Autodesk Fusion 360 part; units mm, degrees
note: some values were not read from the file. Chosen so that the rebuilt part matches the saved one: which bodies a step acts on. Set by a fixed rule: which sketch regions a step uses.
(part 3 of 3)
sketch "Sketch8" plane through (0, 0, -71) normal (0, 0, 1) x (-1, 0, 0) in component "DipCase"
  line L0 (23.45, 45.575) -> (23.45, 72.575)
  arc A0 (18.95, 77.075) -> (23.45, 72.575) centre (23.45, 77.075) ccw
  line L1 (18.95, 77.075) -> (-57.05, 77.075)
  arc A1 (-61.55, 72.575) -> (-57.05, 77.075) centre (-61.55, 77.075) ccw
  line L2 (-61.55, 72.575) -> (-61.55, 66.575)
  line L3 (-61.55, 66.575) -> (-62.84, 66.575)
  line L4 (-62.84, 66.575) -> (-62.84, 51.575)
  line L5 (-62.84, 51.575) -> (-61.55, 51.575)
  line L6 (-61.55, 51.575) -> (-61.55, 45.575)
  arc A2 (-57.05, 41.075) -> (-61.55, 45.575) centre (-61.55, 41.075) ccw
  line L7 (-57.05, 41.075) -> (18.95, 41.075)
  arc A3 (23.45, 45.575) -> (18.95, 41.075) centre (23.45, 41.075) ccw
  line L8 (-61.55, 66.575) -> (-61.55, 51.575)
  constraint coincident L2.end L3.start
  constraint coincident L5.end L6.start
extrude "Extrude7''" add sketch "Sketch8" along normal blind 30 contours L3 L4 L5 L8 bodies 5 in component "DipCase"
sketch "Sketch9" plane through (61.55, 0, 0) normal (-1, 0, 0) x (0, -1, 0) in component "DipCase"
  line L0 (45.575, -71) -> (72.575, -71)
  line L1 (72.575, -71) -> (72.575, -5.6)
  line L2 (72.575, -5.6) -> (66.575, -5.6)
  line L3 (66.575, -5.6) -> (66.575, -41)
  line L4 (66.575, -41) -> (51.575, -41)
  line L5 (51.575, -41) -> (51.575, -5.6)
  line L6 (51.575, -5.6) -> (45.575, -5.6)
  line L7 (45.575, -5.6) -> (45.575, -71)
  line L8 (51.575, -41) -> (45.575, -41)
  line L9 (45.575, -41) -> (66.575, -41)
  line L10 (66.575, -41) -> (72.575, -41)
  line L11 (59.075, -41) -> (59.075, -71) construction
  line L12 (48.075, -51) -> (70.075, -51)
  line L13 (70.075, -51) -> (70.075, -61)
  line L14 (70.075, -61) -> (48.075, -61)
  line L15 (48.075, -61) -> (48.075, -51)
  line L16 (48.075, -51) -> (70.075, -61) construction
  line L17 (70.075, -51) -> (48.075, -61) construction
  line L18 (54.075, -54) -> (64.075, -54)
  line L19 (64.075, -54) -> (64.075, -58)
  line L20 (64.075, -58) -> (54.075, -58)
  line L21 (54.075, -58) -> (54.075, -54)
  line L22 (54.075, -54) -> (64.075, -58) construction
  line L23 (64.075, -54) -> (54.075, -58) construction
  point P0 (59.075, -56)
  point P1 (59.075, -56)
  point P2 (59.075, -56)
  dimension "d257" = 22
  dimension "d258" = 10
  dimension "d259" = 10
  dimension "d260" = 4
  constraint coincident L4.end L5.start
  constraint coincident L7 L8.end
  constraint perpendicular L7 L8
  constraint coincident L3.end L4.start
  constraint coincident L1 L10.end
  constraint perpendicular L1 L10
  constraint midpoint L4 L11.start
  constraint midpoint L0 L11.end
  constraint midpoint L11 P2
  constraint horizontal L12
  constraint perpendicular L12 L13
  constraint parallel L12 L14
  constraint parallel L13 L15
  constraint coincident L16 P2
  constraint coincident L17 P2
  constraint coincident P2 P1
  constraint horizontal L18
  constraint perpendicular L18 L19
  constraint parallel L18 L20
  constraint parallel L19 L21
  constraint coincident L22 P2
  constraint coincident L23 P2
  measures "d257" distance of L13.end L14.end
  measures "d258" distance of L12.end L13.end
  measures "d259" distance of L19.end L20.end
  measures "d260" distance of L18.end L19.end
extrude "Extrude8''" cut sketch "Sketch9" against normal up to surface (5 mm away) contours L18 L19 L20 L21 bodies 5 in component "DipCase"
extrude "Extrude9'" cut sketch "Sketch9" against normal blind 3 contours L12 L13 L14 L15 bodies 5 in component "DipCase"
sketch "Sketch10" plane through (0, -82.075, 0) normal (0, -1, 0) x (1, 0, 0) in component "DipCase"
  line L0 (45.85, -44.8) -> (-7.75, -44.8)
  line L1 (-7.75, -44.8) -> (-7.75, -36.2)
  line L2 (-7.75, -36.2) -> (45.85, -36.2)
  line L3 (45.85, -36.2) -> (45.85, -44.8)
  line L4 (-25.45, -76) -> (63.55, -76)
  line L5 (63.55, -76) -> (63.55, -5.6)
  line L6 (63.55, -5.6) -> (-25.45, -5.6)
  line L7 (-25.45, -5.6) -> (-25.45, -76)
  line L8 (42.85, -41.8) -> (-4.75, -41.8)
  line L9 (-4.75, -41.8) -> (-4.75, -39.2)
  line L10 (-4.75, -39.2) -> (42.85, -39.2)
  line L11 (42.85, -39.2) -> (42.85, -41.8)
  dimension "d268" = 3
extrude "Extrude11" add sketch "Sketch10" against normal up to surface (5 mm away) contours L0 L1 L2 L3 bodies 5 in component "DipCase"
sketch "Sketch1 (5)" plane through (0, -82.075, 0) normal (0, -1, 0) x (1, 0, 0) in component "BusLegend"
  line L0 (-4.75, -39.2) -> (42.85, -39.2)
  line L1 (42.85, -39.2) -> (42.85, -41.8)
  line L2 (42.85, -41.8) -> (-4.75, -41.8)
  line L3 (-4.75, -41.8) -> (-4.75, -39.2)
  line L4 (-25.45, -76) -> (63.55, -76)
  line L5 (63.55, -76) -> (63.55, -5.6)
  line L6 (63.55, -5.6) -> (-25.45, -5.6)
  line L7 (-25.45, -5.6) -> (-25.45, -76)
  line L8 (-4.75, -39.2) -> (42.85, -39.2)
  line L9 (19.05, -39.2) -> (19.05, -41.8) construction
  line L10 (17.78, -40.5) -> (20.32, -40.5) construction
  line L11 (-9.75, -31.2) -> (47.85, -31.2)
  line L12 (47.85, -31.2) -> (47.85, -38.2)
  line L13 (47.85, -38.2) -> (-9.75, -38.2)
  line L14 (-9.75, -38.2) -> (-9.75, -31.2)
  line L15 (-9.75, -31.2) -> (47.85, -38.2) construction
  line L16 (47.85, -31.2) -> (-9.75, -38.2) construction
  line L17 (19.05, -39.2) -> (19.05, -38.2) construction
  line L18 (-4.75, -39.2) -> (-9.75, -39.2) construction
  line L19 (-9.75, -39.2) -> (-9.75, -38.2) construction
  line L20 (-8.75, -37.7) -> (46.85, -37.7) construction
  line L21 (46.85, -37.7) -> (46.85, -31.7) construction
  line L22 (46.85, -31.7) -> (-8.75, -31.7) construction
  line L23 (-8.75, -31.7) -> (-8.75, -37.7) construction
  line L24 (46.85, -37.7) -> (46.85, -37.7001) construction
  line L25 (-8.75, -31.7) -> (46.85, -37.7) construction
  line L26 (-8.75, -37.7) -> (46.85, -31.7) construction
  line L27 (46.85, -31.7) -> (47.85, -31.7) construction
  point P0 (22.86, -40.5)
  point P1 (25.4, -40.5)
  point P2 (27.94, -40.5)
  point P3 (30.48, -40.5)
  point P4 (33.02, -40.5)
  point P5 (35.56, -40.5)
  point P6 (38.1, -40.5)
  point P7 (40.64, -40.5)
  point P8 (15.24, -40.5)
  point P9 (12.7, -40.5)
  point P10 (10.16, -40.5)
  point P11 (7.62, -40.5)
  point P12 (5.08, -40.5)
  point P13 (2.54, -40.5)
  point P14 (0, -40.5)
  point P15 (-2.54, -40.5)
  point P16 (19.05, -34.7)
  point P17 (19.05, -34.7)
  dimension "d272" = 2.54
  dimension "d275" = 2.54
  dimension "d276" = 0
  dimension "d279" = -2.54
  dimension "d280" = 0
  dimension "d281" = 1
  dimension "d282" = 5
  dimension "d283" = 7
  dimension "d284" = 3
  dimension "d285" = 1
  dimension "d286" = 6
  text T0 "GND | MS----------------LS | 5V" font "Arial" height 3 align centre middle in box 55.6 x 6 at (-8.75, -37.7) x (1, 0) y (0, 1) spacing 1
  constraint midpoint L0 L9.start
  constraint midpoint L2 L9.end
  constraint perpendicular L9 L10
  constraint midpoint L9 L10
  constraint horizontal L11
  constraint perpendicular L11 L12
  constraint parallel L11 L13
  constraint parallel L12 L14
  constraint coincident L15 P17
  constraint coincident L16 P17
  constraint midpoint L13 L17.end
  constraint midpoint L15 P17
  constraint perpendicular L13 L17
  constraint coincident L0.start L3.end
  constraint perpendicular L3 L18
  constraint perpendicular L18 L19
  constraint coincident L20.end
  constraint coincident L21 L24.end
  constraint coincident L22.end
  constraint coincident L20.start
  constraint coincident L21.end
  constraint midpoint L26 P17
  constraint horizontal L22
  constraint coincident P17 P16
  constraint coincident L12 L27.end
  constraint perpendicular L12 L27
  measures "d272" distance of L10.start L10.end
  measures "d281" distance of L9.start L17.end
  measures "d282" distance of L0.start L18.end
  measures "d283" distance of L11.end L12.end
  measures "d285" distance of L21.end L27.end
extrude "Extrude1''''" add sketch "Sketch1 (5)" along normal blind 4 separate body text T0 makes body 6 at (-4.9746, -83.4083, -35.2) makes body 7 at (2.3085, -83.4083, -35.7709) makes body 8 at (9.2968, -82.075, -34.7626) makes body 9 at (12.3692, -84.7417, -34.9292) makes body 10 at (15.5377, -83.4083, -35.2996) makes body 11 at (18.329, -83.4083, -35.2996) makes body 12 at (21.1203, -83.4083, -35.2996) makes body 13 at (23.5343, -84.7417, -34.9292) makes body 14 at (26.7028, -84.7417, -35.2996) makes body 15 at (29.1168, -84.7417, -34.9292) makes body 16 at (33.1005, -83.4083, -35.2) makes body 17 at (36.7532, -82.075, -34.7626) makes body 18 at (46.0391, -83.4083, -34.2) makes body 19 at (39.4688, -83.4083, -35.7709) makes body 20 at (41.6735, -83.4083, -34.2682) makes body 21 at (31.9081, -84.7417, -35.2996) makes body 22 at (30.8897, -83.4083, -35.2996) makes body 23 at (28.0984, -83.4083, -35.2996) makes body 24 at (25.3072, -83.4083, -35.2996) makes body 25 at (22.5159, -83.4083, -35.2996) makes body 26 at (19.7246, -83.4083, -35.2996) makes body 27 at (16.5561, -84.7417, -34.9292) makes body 28 at (13.7649, -84.7417, -34.9292) makes body 29 at (11.3508, -83.4083, -35.2996) makes body 30 at (4.4879, -83.4083, -35.2) makes body 31 at (-1.9439, -83.4083, -35.2) makes body 32 at (-6.4029, -84.7417, -34.6707) in component "BusLegend"
extrude "Extrude2''''" add sketch "Sketch1 (5)" along normal blind 3 contours L11 L12 L13 L14 bodies 6 7 8 9 10 11 12 13 14 15 16 17 18 19 20 21 22 23 24 25 26 27 28 29 30 31 32 in component "BusLegend"
sketch "Sketch2 (5)" plane through (0, -85.075, 0) normal (0, -1, 0) x (1, 0, 0) in component "BusLegend"
  line L0 (-9.75, -38.2) -> (47.85, -38.2)
  line L1 (47.85, -38.2) -> (47.85, -31.2)
  line L2 (47.85, -31.2) -> (-9.75, -31.2)
  line L3 (-9.75, -31.2) -> (-9.75, -38.2)
  line L4 (-6.8265, -35.0233) -> (-6.8265, -34.6714)
  line L5 (-6.8265, -34.6714) -> (-5.5557, -34.6693)
  line L6 (-5.5557, -34.6693) -> (-5.5557, -35.7825)
  spline S0 degree 3 poles (-6.1594, -36.1335) (-6.0463, -36.0845) (-5.9446, -36.0405) (-5.7434, -35.9229) (-5.6496, -35.8527) (-5.5557, -35.7825) knots -0.070377 -0.070377 -0.070377 -0.070377 -0.035159 -0.035159 0 0 0 0
  spline S1 degree 3 poles (-6.7979, -36.2512) (-6.6879, -36.2461) (-6.5797, -36.2412) (-6.3669, -36.2019) (-6.2631, -36.1677) (-6.1594, -36.1335) knots -0.065532 -0.065532 -0.065532 -0.065532 -0.032766 -0.032766 0 0 0 0
  spline S2 degree 3 poles (-7.6011, -36.0619) (-7.4683, -36.1204) (-7.3453, -36.1746) (-7.0773, -36.2371) (-6.9376, -36.2441) (-6.7979, -36.2512) knots -0.083967 -0.083967 -0.083967 -0.083967 -0.041966 -0.041966 0 0 0 0
  spline S3 degree 3 poles (-8.1465, -35.5145) (-8.0768, -35.628) (-8.0081, -35.7401) (-7.8262, -35.9225) (-7.7136, -35.9922) (-7.6011, -36.0619) knots -0.079423 -0.079423 -0.079423 -0.079423 -0.039711 -0.039711 0 0 0 0
  spline S4 degree 3 poles (-8.3306, -34.7143) (-8.3239, -34.8533) (-8.3172, -34.9922) (-8.2565, -35.2593) (-8.2039, -35.3813) (-8.1465, -35.5145) knots -0.086964 -0.086964 -0.086964 -0.086964 -0.043506 -0.043506 0 0 0 0
  spline S5 degree 3 poles (-8.1475, -33.8968) (-8.2025, -34.0303) (-8.2554, -34.1587) (-8.3161, -34.4313) (-8.3234, -34.5728) (-8.3306, -34.7143) knots -0.085018 -0.085018 -0.085018 -0.085018 -0.042505 -0.042505 0 0 0 0
  spline S6 degree 3 poles (-7.6205, -33.333) (-7.7355, -33.4081) (-7.8421, -33.4776) (-8.0172, -33.6662) (-8.0823, -33.7815) (-8.1475, -33.8968) knots -0.079495 -0.079495 -0.079495 -0.079495 -0.039731 -0.039731 0 0 0 0
  spline S7 degree 3 poles (-6.8286, -33.1488) (-6.9664, -33.1551) (-7.1042, -33.1614) (-7.3687, -33.2217) (-7.4868, -33.2739) (-7.6205, -33.333) knots -0.087597 -0.087597 -0.087597 -0.087597 -0.043852 -0.043852 0 0 0 0
  spline S8 degree 3 poles (-6.2402, -33.2542) (-6.3414, -33.2205) (-6.4309, -33.1906) (-6.6274, -33.156) (-6.728, -33.1524) (-6.8286, -33.1488) knots -0.060473 -0.060473 -0.060473 -0.060473 -0.030201 -0.030201 0 0 0 0
  spline S9 degree 3 poles (-5.8279, -33.5479) (-5.8908, -33.4808) (-5.9453, -33.4227) (-6.0835, -33.3254) (-6.1619, -33.2898) (-6.2402, -33.2542) knots -0.051721 -0.051721 -0.051721 -0.051721 -0.025816 -0.025816 0 0 0 0
  spline S10 degree 3 poles (-5.6008, -34.039) (-5.626, -33.9512) (-5.6513, -33.8635) (-5.7263, -33.6986) (-5.772, -33.6309) (-5.8279, -33.5479) knots -0.059807 -0.059807 -0.059807 -0.059807 -0.030023 -0.030023 0 0 0 0
  line L7 (-5.6008, -34.039) -> (-5.9589, -34.1372)
  spline S11 degree 3 poles (-6.1267, -33.7771) (-6.0861, -33.8397) (-6.0546, -33.8883) (-5.9991, -34.0097) (-5.979, -34.0735) (-5.9589, -34.1372) knots -0.040416 -0.040416 -0.040416 -0.040416 -0.020059 -0.020059 0 0 0 0
  spline S12 degree 3 poles (-6.4132, -33.5673) (-6.3586, -33.5931) (-6.304, -33.6189) (-6.2078, -33.6884) (-6.1707, -33.729) (-6.1267, -33.7771) knots -0.039026 -0.039026 -0.039026 -0.039026 -0.019563 -0.019563 0 0 0 0
  spline S13 degree 3 poles (-6.8265, -33.4885) (-6.7556, -33.4913) (-6.6847, -33.4941) (-6.5468, -33.52) (-6.4835, -33.5424) (-6.4132, -33.5673) knots -0.044711 -0.044711 -0.044711 -0.044711 -0.022375 -0.022375 0 0 0 0
  spline S14 degree 3 poles (-7.2972, -33.5714) (-7.2141, -33.5434) (-7.1451, -33.5202) (-6.9876, -33.4933) (-6.9071, -33.4909) (-6.8265, -33.4885) knots -0.048493 -0.048493 -0.048493 -0.048493 -0.024168 -0.024168 0 0 0 0
  spline S15 degree 3 poles (-7.6175, -33.7894) (-7.567, -33.7408) (-7.5233, -33.6988) (-7.416, -33.6265) (-7.3566, -33.599) (-7.2972, -33.5714) knots -0.039361 -0.039361 -0.039361 -0.039361 -0.019646 -0.019646 0 0 0 0
  spline S16 degree 3 poles (-7.8068, -34.0861) (-7.7811, -34.0316) (-7.7564, -33.9791) (-7.6932, -33.8802) (-7.6553, -33.8348) (-7.6175, -33.7894) knots -0.035488 -0.035488 -0.035488 -0.035488 -0.017742 -0.017742 0 0 0 0
  spline S17 degree 3 poles (-7.9214, -34.6898) (-7.9171, -34.5863) (-7.9128, -34.4829) (-7.8749, -34.2815) (-7.8421, -34.1874) (-7.8068, -34.0861) knots -0.064337 -0.064337 -0.064337 -0.064337 -0.032181 -0.032181 0 0 0 0
  spline S18 degree 3 poles (-7.7832, -35.361) (-7.831, -35.2426) (-7.8696, -35.147) (-7.9141, -34.9218) (-7.9177, -34.8058) (-7.9214, -34.6898) knots -0.069971 -0.069971 -0.069971 -0.069971 -0.034827 -0.034827 0 0 0 0
  spline S19 degree 3 poles (-7.3811, -35.7621) (-7.466, -35.7111) (-7.5483, -35.6617) (-7.6821, -35.5278) (-7.7327, -35.4444) (-7.7832, -35.361) knots -0.058521 -0.058521 -0.058521 -0.058521 -0.029259 -0.029259 0 0 0 0
  spline S20 degree 3 poles (-6.8204, -35.893) (-6.9177, -35.8876) (-7.015, -35.8822) (-7.2019, -35.8386) (-7.2912, -35.8005) (-7.3811, -35.7621) knots -0.05867 -0.05867 -0.05867 -0.05867 -0.029335 -0.029335 0 0 0 0
  spline S21 degree 3 poles (-6.317, -35.7938) (-6.3985, -35.8225) (-6.48, -35.8513) (-6.6478, -35.8845) (-6.7329, -35.8887) (-6.8204, -35.893) knots -0.052539 -0.052539 -0.052539 -0.052539 -0.026271 -0.026271 0 0 0 0
  spline S22 degree 3 poles (-5.9445, -35.582) (-6.0094, -35.6308) (-6.0582, -35.6677) (-6.1842, -35.738) (-6.2506, -35.7659) (-6.317, -35.7938) knots -0.043642 -0.043642 -0.043642 -0.043642 -0.0216 -0.0216 0 0 0 0
  line L8 (-5.9445, -35.582) -> (-5.9445, -35.0233)
  line L9 (-5.9445, -35.0233) -> (-6.8265, -35.0233)
  line L10 (4.4879, -36.2) -> (4.4879, -33.2)
  line L11 (4.4879, -33.2) -> (5.0855, -33.2)
  line L12 (5.0855, -33.2) -> (5.7956, -35.3241)
  spline S23 degree 3 poles (5.9388, -35.7682) (5.9122, -35.6833) (5.8933, -35.623) (5.8444, -35.4718) (5.82, -35.398) (5.7956, -35.3241) knots -0.047666 -0.047666 -0.047666 -0.047666 -0.023331 -0.023331 0 0 0 0
  spline S24 degree 3 poles (6.0984, -35.2873) (6.0711, -35.3672) (6.0438, -35.4472) (5.9894, -35.6106) (5.9684, -35.6762) (5.9388, -35.7682) knots -0.056865 -0.056865 -0.056865 -0.056865 -0.028983 -0.028983 0 0 0 0
  line L13 (6.0984, -35.2873) -> (6.8167, -33.2)
  line L14 (6.8167, -33.2) -> (7.3508, -33.2)
  line L15 (7.3508, -33.2) -> (7.3508, -36.2)
  line L16 (7.3508, -36.2) -> (6.9681, -36.2)
  line L17 (6.9681, -36.2) -> (6.9681, -33.6891)
  line L18 (6.9681, -33.6891) -> (6.0964, -36.2)
  line L19 (6.0964, -36.2) -> (5.7383, -36.2)
  line L20 (5.7383, -36.2) -> (4.8706, -33.6461)
  line L21 (4.8706, -33.6461) -> (4.8706, -36.2)
  line L22 (4.8706, -36.2) -> (4.4879, -36.2)
  line L23 (13.3877, -35.2996) -> (13.3877, -34.9292)
  line L24 (13.3877, -34.9292) -> (14.5193, -34.9292)
  line L25 (14.5193, -34.9292) -> (14.5193, -35.2996)
  line L26 (14.5193, -35.2996) -> (13.3877, -35.2996)
  line L27 (18.9702, -35.2996) -> (18.9702, -34.9292)
  line L28 (18.9702, -34.9292) -> (20.1018, -34.9292)
  line L29 (20.1018, -34.9292) -> (20.1018, -35.2996)
  line L30 (20.1018, -35.2996) -> (18.9702, -35.2996)
  line L31 (24.5527, -35.2996) -> (24.5527, -34.9292)
  line L32 (24.5527, -34.9292) -> (25.6844, -34.9292)
  line L33 (25.6844, -34.9292) -> (25.6844, -35.2996)
  line L34 (25.6844, -35.2996) -> (24.5527, -35.2996)
  line L35 (30.1353, -35.2996) -> (30.1353, -34.9292)
  line L36 (30.1353, -34.9292) -> (31.2669, -34.9292)
  line L37 (31.2669, -34.9292) -> (31.2669, -35.2996)
  line L38 (31.2669, -35.2996) -> (30.1353, -35.2996)
  line L39 (34.975, -35.846) -> (34.975, -36.2)
  line L40 (34.975, -36.2) -> (33.1005, -36.2)
  line L41 (35.3126, -35.2362) -> (35.6871, -35.2034)
  line L42 (41.9224, -34.8269) -> (41.5766, -34.7819)
  line L43 (41.5766, -34.7819) -> (41.8672, -33.2409)
  spline S25 degree 3 poles (45.2151, -35.3794) (45.1856, -35.4604) (45.1561, -35.5414) (45.1022, -35.7052) (45.0781, -35.7868) (45.0534, -35.8705) knots -0.052408 -0.052408 -0.052408 -0.052408 -0.026205 -0.026205 0 0 0 0
  line L44 (41.8672, -33.2409) -> (43.359, -33.2409)
  line L45 (43.359, -33.2409) -> (43.359, -33.5929)
  line L46 (43.359, -33.5929) -> (42.1619, -33.5929)
  line L47 (42.1619, -33.5929) -> (42.0002, -34.3992)
  line L48 (39.4688, -37.082) -> (39.4688, -33.1488)
  line L49 (39.4688, -33.1488) -> (39.7901, -33.1488)
  line L50 (39.7901, -33.1488) -> (39.7901, -37.082)
  line L51 (37.6107, -34.0452) -> (37.2301, -34.0738)
  line L52 (25.9484, -35.2996) -> (25.9484, -34.9292)
  line L53 (25.9484, -34.9292) -> (27.08, -34.9292)
  line L54 (27.08, -34.9292) -> (27.08, -35.2996)
  line L55 (27.08, -35.2996) -> (25.9484, -35.2996)
  line L56 (20.3658, -35.2996) -> (20.3658, -34.9292)
  line L57 (20.3658, -34.9292) -> (21.4975, -34.9292)
  line L58 (21.4975, -34.9292) -> (21.4975, -35.2996)
  line L59 (21.4975, -35.2996) -> (20.3658, -35.2996)
  line L60 (14.7833, -35.2996) -> (14.7833, -34.9292)
  line L61 (14.7833, -34.9292) -> (15.9149, -34.9292)
  line L62 (15.9149, -34.9292) -> (15.9149, -35.2996)
  line L63 (15.9149, -35.2996) -> (14.7833, -35.2996)
  line L64 (7.8563, -35.2362) -> (8.2308, -35.2034)
  spline S26 degree 3 poles (8.3546, -35.5728) (8.3196, -35.5095) (8.2911, -35.4579) (8.2505, -35.3339) (8.2406, -35.2687) (8.2308, -35.2034) knots -0.039768 -0.039768 -0.039768 -0.039768 -0.019802 -0.019802 0 0 0 0
  spline S27 degree 3 poles (8.6564, -35.8061) (8.5978, -35.7777) (8.5392, -35.7494) (8.4375, -35.6722) (8.4001, -35.6274) (8.3546, -35.5728) knots -0.042533 -0.042533 -0.042533 -0.042533 -0.021347 -0.021347 0 0 0 0
  spline S28 degree 3 poles (9.1168, -35.8951) (9.0378, -35.892) (8.9587, -35.889) (8.805, -35.8598) (8.7352, -35.8346) (8.6564, -35.8061) knots -0.050191 -0.050191 -0.050191 -0.050191 -0.025125 -0.025125 0 0 0 0
  spline S29 degree 3 poles (9.5179, -35.8276) (9.4476, -35.8499) (9.3878, -35.8689) (9.2537, -35.8909) (9.1853, -35.893) (9.1168, -35.8951) knots -0.041174 -0.041174 -0.041174 -0.041174 -0.02054 -0.02054 0 0 0 0
  spline S30 degree 3 poles (9.7768, -35.6424) (9.7372, -35.6867) (9.7048, -35.723) (9.6176, -35.7842) (9.5678, -35.8059) (9.5179, -35.8276) knots -0.032744 -0.032744 -0.032744 -0.032744 -0.016308 -0.016308 0 0 0 0
  spline S31 degree 3 poles (9.8617, -35.3855) (9.8579, -35.4328) (9.8543, -35.478) (9.8258, -35.5635) (9.8013, -35.603) (9.7768, -35.6424) knots -0.027842 -0.027842 -0.027842 -0.027842 -0.013919 -0.013919 0 0 0 0
  spline S32 degree 3 poles (9.7799, -35.1389) (9.8048, -35.1776) (9.8284, -35.214) (9.8554, -35.2963) (9.8586, -35.3409) (9.8617, -35.3855) knots -0.02684 -0.02684 -0.02684 -0.02684 -0.013417 -0.013417 0 0 0 0
  spline S33 degree 3 poles (9.5098, -34.9619) (9.5607, -34.9827) (9.6116, -35.0035) (9.7033, -35.0619) (9.7363, -35.0951) (9.7799, -35.1389) knots -0.036715 -0.036715 -0.036715 -0.036715 -0.018529 -0.018529 0 0 0 0
  spline S34 degree 3 poles (8.9756, -34.8156) (9.0656, -34.8368) (9.1555, -34.858) (9.342, -34.9082) (9.4105, -34.9301) (9.5098, -34.9619) knots -0.059863 -0.059863 -0.059863 -0.059863 -0.031262 -0.031262 0 0 0 0
  spline S35 degree 3 poles (8.3965, -34.6284) (8.5037, -34.6739) (8.5786, -34.7058) (8.7775, -34.7683) (8.8766, -34.792) (8.9756, -34.8156) knots -0.062787 -0.062787 -0.062787 -0.062787 -0.030552 -0.030552 0 0 0 0
  spline S36 degree 3 poles (8.0763, -34.349) (8.1237, -34.4111) (8.1637, -34.4634) (8.2714, -34.5561) (8.3339, -34.5922) (8.3965, -34.6284) knots -0.043479 -0.043479 -0.043479 -0.043479 -0.021682 -0.021682 0 0 0 0
  spline S37 degree 3 poles (7.9709, -33.9756) (7.975, -34.0416) (7.9791, -34.1077) (8.014, -34.2323) (8.0444, -34.2893) (8.0763, -34.349) knots -0.040617 -0.040617 -0.040617 -0.040617 -0.020311 -0.020311 0 0 0 0
  spline S38 degree 3 poles (8.0998, -33.551) (8.0626, -33.617) (8.0253, -33.683) (7.9822, -33.8245) (7.9766, -33.8986) (7.9709, -33.9756) knots -0.04632 -0.04632 -0.04632 -0.04632 -0.023162 -0.023162 0 0 0 0
  spline S39 degree 3 poles (8.4763, -33.2512) (8.4021, -33.2868) (8.3278, -33.3225) (8.2016, -33.4219) (8.1537, -33.4826) (8.0998, -33.551) knots -0.052159 -0.052159 -0.052159 -0.052159 -0.026108 -0.026108 0 0 0 0
  spline S40 degree 3 poles (9.0268, -33.1488) (8.9325, -33.1524) (8.8382, -33.156) (8.6545, -33.1896) (8.5703, -33.2187) (8.4763, -33.2512) knots -0.059585 -0.059585 -0.059585 -0.059585 -0.02982 -0.02982 0 0 0 0
  spline S41 degree 3 poles (9.6151, -33.2563) (9.5127, -33.2209) (9.4251, -33.1906) (9.2284, -33.1556) (9.1276, -33.1522) (9.0268, -33.1488) knots -0.06063 -0.06063 -0.06063 -0.06063 -0.030251 -0.030251 0 0 0 0
  spline S42 degree 3 poles (10.007, -33.5724) (9.9514, -33.5016) (9.9008, -33.4372) (9.7697, -33.3323) (9.6924, -33.2943) (9.6151, -33.2563) knots -0.051699 -0.051699 -0.051699 -0.051699 -0.025832 -0.025832 0 0 0 0
  spline S43 degree 3 poles (10.1544, -34.0452) (10.1461, -33.9612) (10.1379, -33.8773) (10.0891, -33.7196) (10.0492, -33.6481) (10.007, -33.5724) knots -0.051952 -0.051952 -0.051952 -0.051952 -0.025982 -0.025982 0 0 0 0
  line L65 (10.1544, -34.0452) -> (9.7737, -34.0738)
  spline S44 degree 3 poles (9.566, -33.6441) (9.6279, -33.7102) (9.679, -33.7649) (9.7468, -33.9095) (9.7603, -33.9916) (9.7737, -34.0738) knots -0.050133 -0.050133 -0.050133 -0.050133 -0.024981 -0.024981 0 0 0 0
  spline S45 degree 3 poles (9.0432, -33.4988) (9.1368, -33.5014) (9.2304, -33.5039) (9.4073, -33.55) (9.4756, -33.5905) (9.566, -33.6441) knots -0.062461 -0.062461 -0.062461 -0.062461 -0.031541 -0.031541 0 0 0 0
  spline S46 degree 3 poles (8.5183, -33.6308) (8.6109, -33.5799) (8.6782, -33.5429) (8.8568, -33.5016) (8.95, -33.5002) (9.0432, -33.4988) knots -0.056785 -0.056785 -0.056785 -0.056785 -0.027956 -0.027956 0 0 0 0
  spline S47 degree 3 poles (8.3535, -33.949) (8.3621, -33.8823) (8.3697, -33.8235) (8.4256, -33.7177) (8.4719, -33.6742) (8.5183, -33.6308) knots -0.038169 -0.038169 -0.038169 -0.038169 -0.019061 -0.019061 0 0 0 0
  spline S48 degree 3 poles (8.4702, -34.215) (8.4352, -34.1766) (8.4015, -34.1395) (8.3628, -34.0507) (8.3582, -33.9998) (8.3535, -33.949) knots -0.030649 -0.030649 -0.030649 -0.030649 -0.015323 -0.015323 0 0 0 0
  spline S49 degree 3 poles (9.0688, -34.4289) (8.9637, -34.4069) (8.8586, -34.3849) (8.648, -34.3141) (8.5754, -34.2736) (8.4702, -34.215) knots -0.069078 -0.069078 -0.069078 -0.069078 -0.036122 -0.036122 0 0 0 0
  spline S50 degree 3 poles (9.7328, -34.6202) (9.609, -34.5749) (9.5232, -34.5435) (9.2941, -34.4792) (9.1814, -34.454) (9.0688, -34.4289) knots -0.071539 -0.071539 -0.071539 -0.071539 -0.034637 -0.034637 0 0 0 0
  spline S51 degree 3 poles (10.1196, -34.9261) (10.0609, -34.8554) (10.0129, -34.7976) (9.8826, -34.6962) (9.8077, -34.6582) (9.7328, -34.6202) knots -0.050607 -0.050607 -0.050607 -0.050607 -0.025203 -0.025203 0 0 0 0
  spline S52 degree 3 poles (10.2444, -35.3528) (10.2398, -35.2769) (10.2351, -35.201) (10.1939, -35.0586) (10.1582, -34.9949) (10.1196, -34.9261) knots -0.047283 -0.047283 -0.047283 -0.047283 -0.023651 -0.023651 0 0 0 0
  spline S53 degree 3 poles (10.1073, -35.804) (10.1467, -35.7338) (10.1862, -35.6636) (10.2322, -35.5133) (10.2381, -35.4351) (10.2444, -35.3528) knots -0.049538 -0.049538 -0.049538 -0.049538 -0.024774 -0.024774 0 0 0 0
  spline S54 degree 3 poles (9.7134, -36.1335) (9.7909, -36.0927) (9.8685, -36.0519) (10.0004, -35.9425) (10.051, -35.8769) (10.1073, -35.804) knots -0.055202 -0.055202 -0.055202 -0.055202 -0.027624 -0.027624 0 0 0 0
  spline S55 degree 3 poles (9.1353, -36.2512) (9.2348, -36.2471) (9.3344, -36.243) (9.5274, -36.2044) (9.6151, -36.171) (9.7134, -36.1335) knots -0.063062 -0.063062 -0.063062 -0.063062 -0.031564 -0.031564 0 0 0 0
  spline S56 degree 3 poles (8.4528, -36.1325) (8.5751, -36.174) (8.6727, -36.2071) (8.9017, -36.2452) (9.0185, -36.2482) (9.1353, -36.2512) knots -0.070479 -0.070479 -0.070479 -0.070479 -0.035054 -0.035054 0 0 0 0
  spline S57 degree 3 poles (8.021, -35.7754) (8.081, -35.853) (8.138, -35.9268) (8.2822, -36.0456) (8.3675, -36.089) (8.4528, -36.1325) knots -0.057452 -0.057452 -0.057452 -0.057452 -0.028721 -0.028721 0 0 0 0
  spline S58 degree 3 poles (7.8563, -35.2362) (7.8647, -35.3319) (7.8731, -35.4276) (7.9277, -35.6075) (7.9731, -35.6892) (8.021, -35.7754) knots -0.05915 -0.05915 -0.05915 -0.05915 -0.029581 -0.029581 0 0 0 0
  line L66 (-4.9746, -36.2) -> (-4.9746, -33.2)
  line L67 (-4.9746, -33.2) -> (-4.5673, -33.2)
  line L68 (-4.5673, -33.2) -> (-2.9916, -35.5554)
  line L69 (-2.9916, -35.5554) -> (-2.9916, -33.2)
  line L70 (-2.9916, -33.2) -> (-2.611, -33.2)
  line L71 (-2.611, -33.2) -> (-2.611, -36.2)
  line L72 (-2.611, -36.2) -> (-3.0182, -36.2)
  line L73 (-3.0182, -36.2) -> (-4.5939, -33.8426)
  line L74 (-4.5939, -33.8426) -> (-4.5939, -36.2)
  line L75 (-4.5939, -36.2) -> (-4.9746, -36.2)
  line L76 (2.3085, -37.082) -> (2.3085, -33.1488)
  line L77 (2.3085, -33.1488) -> (2.6298, -33.1488)
  line L78 (2.6298, -33.1488) -> (2.6298, -37.082)
  line L79 (2.6298, -37.082) -> (2.3085, -37.082)
  line L80 (11.992, -35.2996) -> (11.992, -34.9292)
  line L81 (11.992, -34.9292) -> (13.1237, -34.9292)
  line L82 (13.1237, -34.9292) -> (13.1237, -35.2996)
  line L83 (13.1237, -35.2996) -> (11.992, -35.2996)
  line L84 (17.5746, -35.2996) -> (17.5746, -34.9292)
  line L85 (17.5746, -34.9292) -> (18.7062, -34.9292)
  line L86 (18.7062, -34.9292) -> (18.7062, -35.2996)
  line L87 (18.7062, -35.2996) -> (17.5746, -35.2996)
  line L88 (23.1571, -35.2996) -> (23.1571, -34.9292)
  line L89 (23.1571, -34.9292) -> (24.2887, -34.9292)
  line L90 (24.2887, -34.9292) -> (24.2887, -35.2996)
  line L91 (24.2887, -35.2996) -> (23.1571, -35.2996)
  line L92 (28.7396, -35.2996) -> (28.7396, -34.9292)
  line L93 (28.7396, -34.9292) -> (29.8713, -34.9292)
  line L94 (29.8713, -34.9292) -> (29.8713, -35.2996)
  line L95 (29.8713, -35.2996) -> (28.7396, -35.2996)
  line L96 (33.1005, -36.2) -> (33.1005, -33.2)
  line L97 (33.1005, -33.2) -> (33.4975, -33.2)
  line L98 (33.4975, -33.2) -> (33.4975, -35.846)
  line L99 (33.4975, -35.846) -> (34.975, -35.846)
  line L100 (44.8488, -36.2) -> (43.6864, -33.2)
  line L101 (43.6864, -33.2) -> (44.1162, -33.2)
  line L102 (44.1162, -33.2) -> (44.8958, -35.3794)
  line L103 (39.7901, -37.082) -> (39.4688, -37.082)
  line L104 (41.5111, -35.4142) -> (41.8979, -35.3814)
  line L105 (31.5309, -35.2996) -> (31.5309, -34.9292)
  line L106 (31.5309, -34.9292) -> (32.6626, -34.9292)
  line L107 (32.6626, -34.9292) -> (32.6626, -35.2996)
  line L108 (32.6626, -35.2996) -> (31.5309, -35.2996)
  line L109 (27.344, -35.2996) -> (27.344, -34.9292)
  line L110 (27.344, -34.9292) -> (28.4756, -34.9292)
  line L111 (28.4756, -34.9292) -> (28.4756, -35.2996)
  line L112 (28.4756, -35.2996) -> (27.344, -35.2996)
  line L113 (21.7615, -35.2996) -> (21.7615, -34.9292)
  line L114 (21.7615, -34.9292) -> (22.8931, -34.9292)
  line L115 (22.8931, -34.9292) -> (22.8931, -35.2996)
  line L116 (22.8931, -35.2996) -> (21.7615, -35.2996)
  line L117 (16.1789, -35.2996) -> (16.1789, -34.9292)
  line L118 (16.1789, -34.9292) -> (17.3106, -34.9292)
  line L119 (17.3106, -34.9292) -> (17.3106, -35.2996)
  line L120 (17.3106, -35.2996) -> (16.1789, -35.2996)
  line L121 (10.5964, -35.2996) -> (10.5964, -34.9292)
  line L122 (10.5964, -34.9292) -> (11.728, -34.9292)
  line L123 (11.728, -34.9292) -> (11.728, -35.2996)
  line L124 (11.728, -35.2996) -> (10.5964, -35.2996)
  line L125 (-1.9439, -36.2) -> (-1.9439, -33.2)
  line L126 (-1.9439, -33.2) -> (-0.9104, -33.2)
  spline S59 degree 3 poles (-0.3763, -33.243) (-0.4772, -33.2262) (-0.55, -33.2141) (-0.7312, -33.2007) (-0.8208, -33.2004) (-0.9104, -33.2) knots -0.054709 -0.054709 -0.054709 -0.054709 -0.026886 -0.026886 0 0 0 0
  spline S60 degree 3 poles (0.0636, -33.4578) (-0.0061, -33.4062) (-0.0696, -33.3592) (-0.2166, -33.288) (-0.2964, -33.2655) (-0.3763, -33.243) knots -0.049826 -0.049826 -0.049826 -0.049826 -0.024897 -0.024897 0 0 0 0
  spline S61 degree 3 poles (0.4187, -33.9705) (0.376, -33.8735) (0.3334, -33.7766) (0.2154, -33.6054) (0.1421, -33.5341) (0.0636, -33.4578) knots -0.065641 -0.065641 -0.065641 -0.065641 -0.032832 -0.032832 0 0 0 0
  spline S62 degree 3 poles (0.5364, -34.6836) (0.5326, -34.5621) (0.5289, -34.4405) (0.4905, -34.2022) (0.4574, -34.0952) (0.4187, -33.9705) knots -0.078207 -0.078207 -0.078207 -0.078207 -0.039183 -0.039183 0 0 0 0
  spline S63 degree 3 poles (0.4565, -35.2894) (0.4832, -35.1817) (0.5056, -35.091) (0.5315, -34.8885) (0.5339, -34.7861) (0.5364, -34.6836) knots -0.061641 -0.061641 -0.061641 -0.061641 -0.030739 -0.030739 0 0 0 0
  spline S64 degree 3 poles (0.2519, -35.7263) (0.2993, -35.6513) (0.3382, -35.5899) (0.406, -35.4434) (0.4312, -35.3664) (0.4565, -35.2894) knots -0.048813 -0.048813 -0.048813 -0.048813 -0.024315 -0.024315 0 0 0 0
  spline S65 degree 3 poles (-0.0213, -35.9984) (0.0341, -35.9565) (0.0819, -35.9203) (0.1728, -35.8291) (0.2123, -35.7777) (0.2519, -35.7263) knots -0.038992 -0.038992 -0.038992 -0.038992 -0.019459 -0.019459 0 0 0 0
  spline S66 degree 3 poles (-0.3794, -36.1488) (-0.3164, -36.1315) (-0.2535, -36.1142) (-0.1336, -36.0644) (-0.0819, -36.034) (-0.0213, -35.9984) knots -0.042066 -0.042066 -0.042066 -0.042066 -0.021078 -0.021078 0 0 0 0
  spline S67 degree 3 poles (-0.8613, -36.2) (-0.7802, -36.1985) (-0.6991, -36.197) (-0.538, -36.1804) (-0.4659, -36.1661) (-0.3794, -36.1488) knots -0.052738 -0.052738 -0.052738 -0.052738 -0.026449 -0.026449 0 0 0 0
  line L127 (-0.8613, -36.2) -> (-1.9439, -36.2)
  line L128 (-1.5469, -35.846) -> (-0.9063, -35.846)
  spline S68 degree 3 poles (-0.4408, -35.7907) (-0.5276, -35.8116) (-0.5916, -35.827) (-0.749, -35.8444) (-0.8277, -35.8452) (-0.9063, -35.846) knots -0.047822 -0.047822 -0.047822 -0.047822 -0.023604 -0.023604 0 0 0 0
  spline S69 degree 3 poles (-0.1717, -35.6352) (-0.2153, -35.6722) (-0.2517, -35.703) (-0.342, -35.7544) (-0.3914, -35.7726) (-0.4408, -35.7907) knots -0.031681 -0.031681 -0.031681 -0.031681 -0.015792 -0.015792 0 0 0 0
  spline S70 degree 3 poles (0.0483, -35.2556) (0.0225, -35.3253) (-0.0033, -35.3949) (-0.076, -35.5224) (-0.1195, -35.5736) (-0.1717, -35.6352) knots -0.048313 -0.048313 -0.048313 -0.048313 -0.024232 -0.024232 0 0 0 0
  spline S71 degree 3 poles (0.1271, -34.6775) (0.1251, -34.7754) (0.1231, -34.8734) (0.0977, -35.0672) (0.0757, -35.151) (0.0483, -35.2556) knots -0.064561 -0.064561 -0.064561 -0.064561 -0.032443 -0.032443 0 0 0 0
  spline S72 degree 3 poles (-0.0274, -33.9541) (0.0304, -34.084) (0.0734, -34.1809) (0.1222, -34.4256) (0.1247, -34.5515) (0.1271, -34.6775) knots -0.07646 -0.07646 -0.07646 -0.07646 -0.037791 -0.037791 0 0 0 0
  spline S73 degree 3 poles (-0.4029, -33.6154) (-0.3192, -33.6593) (-0.2497, -33.6958) (-0.1252, -33.8102) (-0.0763, -33.8821) (-0.0274, -33.9541) knots -0.05236 -0.05236 -0.05236 -0.05236 -0.026096 -0.026096 0 0 0 0
  spline S74 degree 3 poles (-0.9166, -33.554) (-0.8296, -33.5541) (-0.7426, -33.5543) (-0.5671, -33.5732) (-0.4992, -33.5907) (-0.4029, -33.6154) knots -0.058316 -0.058316 -0.058316 -0.058316 -0.029826 -0.029826 0 0 0 0
  line L129 (-0.9166, -33.554) -> (-1.5469, -33.554)
  line L130 (-1.5469, -33.554) -> (-1.5469, -35.846)
  spline S75 degree 3 poles (42.0974, -35.8061) (42.0396, -35.7378) (41.9938, -35.6836) (41.9286, -35.5404) (41.9133, -35.4609) (41.8979, -35.3814) knots -0.048849 -0.048849 -0.048849 -0.048849 -0.024287 -0.024287 0 0 0 0
  spline S76 degree 3 poles (42.475, -35.9483) (42.4052, -35.9427) (42.3353, -35.9372) (42.2094, -35.89) (42.1547, -35.849) (42.0974, -35.8061) knots -0.042947 -0.042947 -0.042947 -0.042947 -0.021476 -0.021476 0 0 0 0
  spline S77 degree 3 poles (42.9252, -35.7477) (42.8611, -35.8059) (42.797, -35.864) (42.647, -35.931) (42.5621, -35.9396) (42.475, -35.9483) knots -0.052542 -0.052542 -0.052542 -0.052542 -0.026272 -0.026272 0 0 0 0
  spline S78 degree 3 poles (43.1093, -35.2157) (43.1038, -35.3134) (43.0982, -35.411) (43.0384, -35.5895) (42.9866, -35.6618) (42.9252, -35.7477) knots -0.063232 -0.063232 -0.063232 -0.063232 -0.0317 -0.0317 0 0 0 0
  spline S79 degree 3 poles (42.9323, -34.7184) (42.9921, -34.7985) (43.0417, -34.8649) (43.0991, -35.0319) (43.1042, -35.1238) (43.1093, -35.2157) knots -0.055397 -0.055397 -0.055397 -0.055397 -0.027609 -0.027609 0 0 0 0
  spline S80 degree 3 poles (42.4688, -34.5363) (42.5557, -34.5426) (42.6426, -34.5489) (42.7977, -34.6086) (42.8611, -34.6603) (42.9323, -34.7184) knots -0.055105 -0.055105 -0.055105 -0.055105 -0.027582 -0.027582 0 0 0 0
  spline S81 degree 3 poles (42.1475, -34.6171) (42.2003, -34.5921) (42.2492, -34.569) (42.3564, -34.5423) (42.4126, -34.5393) (42.4688, -34.5363) knots -0.033787 -0.033787 -0.033787 -0.033787 -0.016887 -0.016887 0 0 0 0
  spline S82 degree 3 poles (41.9224, -34.8269) (41.9544, -34.7834) (41.9842, -34.7428) (42.0594, -34.6731) (42.1035, -34.6451) (42.1475, -34.6171) knots -0.031324 -0.031324 -0.031324 -0.031324 -0.015657 -0.015657 0 0 0 0
  spline S83 degree 3 poles (42.5671, -34.2109) (42.4603, -34.2203) (42.3636, -34.2288) (42.1747, -34.2924) (42.0875, -34.3458) (42.0002, -34.3992) knots -0.061432 -0.061432 -0.061432 -0.061432 -0.030694 -0.030694 0 0 0 0
  spline S84 degree 3 poles (43.2301, -34.4831) (43.1326, -34.4021) (43.0376, -34.3232) (42.8164, -34.2328) (42.6917, -34.2219) (42.5671, -34.2109) knots -0.075104 -0.075104 -0.075104 -0.075104 -0.03755 -0.03755 0 0 0 0
  spline S85 degree 3 poles (43.5002, -35.1829) (43.4907, -35.0523) (43.4812, -34.9217) (43.3924, -34.6877) (43.3156, -34.5909) (43.2301, -34.4831) knots -0.08248 -0.08248 -0.08248 -0.08248 -0.041276 -0.041276 0 0 0 0
  spline S86 degree 3 poles (43.2628, -35.8869) (43.3358, -35.7765) (43.4039, -35.6735) (43.4823, -35.4385) (43.4912, -35.3107) (43.5002, -35.1829) knots -0.076871 -0.076871 -0.076871 -0.076871 -0.038422 -0.038422 0 0 0 0
  spline S87 degree 3 poles (42.475, -36.2512) (42.6284, -36.2376) (42.7817, -36.224) (43.0451, -36.1038) (43.1498, -35.9995) (43.2628, -35.8869) knots -0.095684 -0.095684 -0.095684 -0.095684 -0.047862 -0.047862 0 0 0 0
  spline S88 degree 3 poles (41.8068, -36.022) (41.9143, -36.0972) (42.0067, -36.1618) (42.2304, -36.2365) (42.3527, -36.2439) (42.475, -36.2512) knots -0.07363 -0.07363 -0.07363 -0.07363 -0.036743 -0.036743 0 0 0 0
  spline S89 degree 3 poles (41.5111, -35.4142) (41.5309, -35.53) (41.5507, -35.6458) (41.6484, -35.8491) (41.7239, -35.9314) (41.8068, -36.022) knots -0.073626 -0.073626 -0.073626 -0.073626 -0.036838 -0.036838 0 0 0 0
  spline S90 degree 3 poles (45.0534, -35.8705) (45.0279, -35.7826) (45.0056, -35.7056) (44.9529, -35.5417) (44.9244, -35.4605) (44.8958, -35.3794) knots -0.051674 -0.051674 -0.051674 -0.051674 -0.0258 -0.0258 0 0 0 0
  line L131 (45.2151, -35.3794) -> (46.0254, -33.2)
  line L132 (46.0254, -33.2) -> (46.4306, -33.2)
  line L133 (46.4306, -33.2) -> (45.256, -36.2)
  line L134 (45.256, -36.2) -> (44.8488, -36.2)
  spline S91 degree 3 poles (35.8109, -35.5728) (35.7759, -35.5095) (35.7474, -35.4579) (35.7069, -35.3339) (35.697, -35.2687) (35.6871, -35.2034) knots -0.039768 -0.039768 -0.039768 -0.039768 -0.019802 -0.019802 0 0 0 0
  spline S92 degree 3 poles (36.1128, -35.8061) (36.0541, -35.7777) (35.9955, -35.7494) (35.8938, -35.6722) (35.8565, -35.6274) (35.8109, -35.5728) knots -0.042533 -0.042533 -0.042533 -0.042533 -0.021347 -0.021347 0 0 0 0
  spline S93 degree 3 poles (36.5732, -35.8951) (36.4941, -35.892) (36.4151, -35.889) (36.2613, -35.8598) (36.1915, -35.8346) (36.1128, -35.8061) knots -0.050191 -0.050191 -0.050191 -0.050191 -0.025124 -0.025124 0 0 0 0
  spline S94 degree 3 poles (36.9743, -35.8276) (36.904, -35.8499) (36.8442, -35.8689) (36.7101, -35.8909) (36.6416, -35.893) (36.5732, -35.8951) knots -0.041174 -0.041174 -0.041174 -0.041174 -0.02054 -0.02054 0 0 0 0
  spline S95 degree 3 poles (37.2332, -35.6424) (37.1936, -35.6867) (37.1612, -35.723) (37.074, -35.7842) (37.0241, -35.8059) (36.9743, -35.8276) knots -0.032744 -0.032744 -0.032744 -0.032744 -0.016308 -0.016308 0 0 0 0
  spline S96 degree 3 poles (37.3181, -35.3855) (37.3143, -35.4328) (37.3106, -35.478) (37.2821, -35.5635) (37.2576, -35.603) (37.2332, -35.6424) knots -0.027842 -0.027842 -0.027842 -0.027842 -0.013919 -0.013919 0 0 0 0
  spline S97 degree 3 poles (37.2362, -35.1389) (37.2612, -35.1776) (37.2847, -35.214) (37.3118, -35.2963) (37.3149, -35.3409) (37.3181, -35.3855) knots -0.02684 -0.02684 -0.02684 -0.02684 -0.013417 -0.013417 0 0 0 0
  spline S98 degree 3 poles (36.9661, -34.9619) (37.017, -34.9827) (37.068, -35.0035) (37.1596, -35.0619) (37.1927, -35.0951) (37.2362, -35.1389) knots -0.036714 -0.036714 -0.036714 -0.036714 -0.018529 -0.018529 0 0 0 0
  spline S99 degree 3 poles (36.432, -34.8156) (36.5219, -34.8368) (36.6118, -34.858) (36.7984, -34.9082) (36.8669, -34.9301) (36.9661, -34.9619) knots -0.059863 -0.059863 -0.059863 -0.059863 -0.031262 -0.031262 0 0 0 0
  spline S100 degree 3 poles (35.8529, -34.6284) (35.9601, -34.6739) (36.035, -34.7058) (36.2339, -34.7683) (36.3329, -34.792) (36.432, -34.8156) knots -0.062787 -0.062787 -0.062787 -0.062787 -0.030552 -0.030552 0 0 0 0
  spline S101 degree 3 poles (35.5326, -34.349) (35.5801, -34.4111) (35.62, -34.4634) (35.7277, -34.5561) (35.7903, -34.5922) (35.8529, -34.6284) knots -0.04348 -0.04348 -0.04348 -0.04348 -0.021682 -0.021682 0 0 0 0
  spline S102 degree 3 poles (35.4272, -33.9756) (35.4313, -34.0416) (35.4355, -34.1077) (35.4704, -34.2323) (35.5008, -34.2893) (35.5326, -34.349) knots -0.040617 -0.040617 -0.040617 -0.040617 -0.020311 -0.020311 0 0 0 0
  spline S103 degree 3 poles (35.5561, -33.551) (35.5189, -33.617) (35.4817, -33.683) (35.4385, -33.8245) (35.433, -33.8986) (35.4272, -33.9756) knots -0.04632 -0.04632 -0.04632 -0.04632 -0.023162 -0.023162 0 0 0 0
  spline S104 degree 3 poles (35.9327, -33.2512) (35.8584, -33.2868) (35.7841, -33.3225) (35.658, -33.4219) (35.6101, -33.4826) (35.5561, -33.551) knots -0.05216 -0.05216 -0.05216 -0.05216 -0.026108 -0.026108 0 0 0 0
  spline S105 degree 3 poles (36.4832, -33.1488) (36.3889, -33.1524) (36.2946, -33.156) (36.1108, -33.1896) (36.0266, -33.2187) (35.9327, -33.2512) knots -0.059584 -0.059584 -0.059584 -0.059584 -0.02982 -0.02982 0 0 0 0
  spline S106 degree 3 poles (37.0715, -33.2563) (36.969, -33.2209) (36.8814, -33.1906) (36.6847, -33.1556) (36.5839, -33.1522) (36.4832, -33.1488) knots -0.06063 -0.06063 -0.06063 -0.06063 -0.030251 -0.030251 0 0 0 0
  spline S107 degree 3 poles (37.4634, -33.5724) (37.4077, -33.5016) (37.3571, -33.4372) (37.226, -33.3323) (37.1487, -33.2943) (37.0715, -33.2563) knots -0.051699 -0.051699 -0.051699 -0.051699 -0.025832 -0.025832 0 0 0 0
  spline S108 degree 3 poles (37.6107, -34.0452) (37.6025, -33.9612) (37.5943, -33.8773) (37.5455, -33.7196) (37.5056, -33.6481) (37.4634, -33.5724) knots -0.051952 -0.051952 -0.051952 -0.051952 -0.025982 -0.025982 0 0 0 0
  spline S109 degree 3 poles (37.0224, -33.6441) (37.0842, -33.7102) (37.1353, -33.7649) (37.2031, -33.9095) (37.2166, -33.9916) (37.2301, -34.0738) knots -0.050134 -0.050134 -0.050134 -0.050134 -0.024981 -0.024981 0 0 0 0
  spline S110 degree 3 poles (36.4995, -33.4988) (36.5931, -33.5014) (36.6867, -33.5039) (36.8636, -33.55) (36.9319, -33.5905) (37.0224, -33.6441) knots -0.062461 -0.062461 -0.062461 -0.062461 -0.031541 -0.031541 0 0 0 0
  spline S111 degree 3 poles (35.9746, -33.6308) (36.0672, -33.5799) (36.1345, -33.5429) (36.3132, -33.5016) (36.4064, -33.5002) (36.4995, -33.4988) knots -0.056785 -0.056785 -0.056785 -0.056785 -0.027956 -0.027956 0 0 0 0
  spline S112 degree 3 poles (35.8099, -33.949) (35.8185, -33.8823) (35.8261, -33.8235) (35.8819, -33.7177) (35.9283, -33.6742) (35.9746, -33.6308) knots -0.038169 -0.038169 -0.038169 -0.038169 -0.019061 -0.019061 0 0 0 0
  spline S113 degree 3 poles (35.9265, -34.215) (35.8916, -34.1766) (35.8579, -34.1395) (35.8192, -34.0507) (35.8145, -33.9998) (35.8099, -33.949) knots -0.030649 -0.030649 -0.030649 -0.030649 -0.015323 -0.015323 0 0 0 0
  spline S114 degree 3 poles (36.5251, -34.4289) (36.42, -34.4069) (36.3149, -34.3849) (36.1043, -34.3141) (36.0317, -34.2736) (35.9265, -34.215) knots -0.069078 -0.069078 -0.069078 -0.069078 -0.036122 -0.036122 0 0 0 0
  spline S115 degree 3 poles (37.1892, -34.6202) (37.0654, -34.5749) (36.9795, -34.5435) (36.7505, -34.4792) (36.6378, -34.454) (36.5251, -34.4289) knots -0.071539 -0.071539 -0.071539 -0.071539 -0.034637 -0.034637 0 0 0 0
  spline S116 degree 3 poles (37.5759, -34.9261) (37.5172, -34.8554) (37.4693, -34.7976) (37.339, -34.6962) (37.2641, -34.6582) (37.1892, -34.6202) knots -0.050607 -0.050607 -0.050607 -0.050607 -0.025203 -0.025203 0 0 0 0
  spline S117 degree 3 poles (37.7007, -35.3528) (37.6961, -35.2769) (37.6914, -35.201) (37.6503, -35.0586) (37.6145, -34.9949) (37.5759, -34.9261) knots -0.047283 -0.047283 -0.047283 -0.047283 -0.023651 -0.023651 0 0 0 0
  spline S118 degree 3 poles (37.5636, -35.804) (37.6031, -35.7338) (37.6425, -35.6636) (37.6885, -35.5133) (37.6945, -35.4351) (37.7007, -35.3528) knots -0.049538 -0.049538 -0.049538 -0.049538 -0.024774 -0.024774 0 0 0 0
  spline S119 degree 3 poles (37.1697, -36.1335) (37.2473, -36.0927) (37.3248, -36.0519) (37.4567, -35.9425) (37.5074, -35.8769) (37.5636, -35.804) knots -0.055202 -0.055202 -0.055202 -0.055202 -0.027624 -0.027624 0 0 0 0
  spline S120 degree 3 poles (36.5916, -36.2512) (36.6912, -36.2471) (36.7908, -36.243) (36.9838, -36.2044) (37.0714, -36.171) (37.1697, -36.1335) knots -0.063062 -0.063062 -0.063062 -0.063062 -0.031564 -0.031564 0 0 0 0
  spline S121 degree 3 poles (35.9091, -36.1325) (36.0314, -36.174) (36.129, -36.2071) (36.358, -36.2452) (36.4748, -36.2482) (36.5916, -36.2512) knots -0.070479 -0.070479 -0.070479 -0.070479 -0.035053 -0.035053 0 0 0 0
  spline S122 degree 3 poles (35.4774, -35.7754) (35.5373, -35.853) (35.5943, -35.9268) (35.7385, -36.0456) (35.8238, -36.089) (35.9091, -36.1325) knots -0.057452 -0.057452 -0.057452 -0.057452 -0.028721 -0.028721 0 0 0 0
  spline S123 degree 3 poles (35.3126, -35.2362) (35.321, -35.3319) (35.3294, -35.4276) (35.384, -35.6075) (35.4294, -35.6892) (35.4774, -35.7754) knots -0.05915 -0.05915 -0.05915 -0.05915 -0.029581 -0.029581 0 0 0 0
component "Plate" placed x (1, 0, 0) y (0, 1, 0) z (0, 0, 1) at (0, 0, 0)
component "Case" placed x (1, 0, 0) y (0, 1, 0) z (0, 0, 1) at (0, 0, 0)
component "DipPlate" placed x (-1, 0, 0) y (0, -1, 0) z (0, 0, 1) at (17.84, -59.075, -5.6)
component "DipCase" placed x (1, 0, 0) y (0, 1, 0) z (0, 0, 1) at (0, 0, 0)
component "BusLegend" placed x (1, 0, 0) y (0, 1, 0) z (0, 0, 1) at (0, 0, 0)
component "Insert" placed x (1, 0, 0) y (0, 1, 0) z (0, 0, 1) at (0, 0, 0) in component "Plate"
equation "WallThickness = 5 mm"
equation "d24 = 80 mm + ( WallThickness * 2 ) + 5 mm"
equation "d25 = WallThickness * 2"
equation "d32 = M3HoleDiameter"
equation "d35 = WallThickness * 2"
equation "d100 = -WallThickness"
equation "M3InsertDiameter = 4.6 mm"
equation "M3InsertLength = 6 mm"
equation "d103 = M3InsertDiameter"
equation "d105 = M3InsertLength"
equation "d109 = WallThickness"
equation "d118 = 68 mm - 2.19 mm"
equation "d119 = 28.18 mm - 2.19 mm"
equation "M1p6InsertDiameter = 2.3 mm"
equation "M1p6InsertLength = 4 mm"
equation "d122 = M1p6InsertDiameter"
equation "d124 = M3InsertLength"
equation "d126 = M1p6InsertLength + 16 mm"
equation "d143 = 68 mm - 2.19 mm"
equation "d144 = 28.18 mm - 2.19 mm"
equation "d145 = M1p6InsertDiameter"
equation "d148 = M1p6InsertDiameter"
equation "d149 = -M1p6InsertLength"
equation "d152 = M3HoleDiameter"
equation "d161 = M1p6InsertDiameter"
equation "d168 = 5.35 mm + 27.94 mm + 0.5 mm"
equation "d173 = 3 mm + WallThickness"
equation "d214 = M1p6InsertLength"
equation "d216 = -WallThickness"
equation "M3HoleDiameter = 4 mm"
equation "d219 = M3HoleDiameter"
equation "d230 = -WallThickness"
equation "d233 = M3InsertDiameter"
equation "d250 = M3InsertDiameter"
equation "d263 = -WallThickness + 2 mm"
equation "d265 = M3InsertLength"
